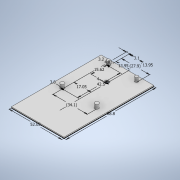
# Autodesk Inventor part: test fit for rfid reader
Saved by Autodesk Inventor 2020 (Build 240168000, 168)
## iProperties
Created: 2019-06-28
Part Number: test fit for rfid reader
Material: Generic
Document SubType Name: Modeling
Designer: jjsch
Density: 1 g/cm^3
Appearance: Default
Author: jjsch
Autodesk Inventor part; units mm, degrees
ref_plane "YZ Plane" through (0, 0, 0) normal (1, 0, 0) x (0, 1, 0)
ref_plane "XZ Plane" through (0, 0, 0) normal (0, 1, 0) x (-1, 0, 0)
ref_plane "XY Plane" through (0, 0, 0) normal (0, 0, 1) x (1, 0, 0)
sketch "Sketch1" plane through (0, 0, 0) normal (0, 1, 0) x (-1, 0, 0)
  point P0 (0, 0)
sketch "Sketch2" plane through (0, 0, 0) normal (0, 1, 0) x (-1, 0, 0)
  line L0 (0, 0) -> (-52.05, 0)
  line L1 (-52.05, 0) -> (-52.05, 88.8)
  line L2 (-52.05, 88.8) -> (0, 88.8)
  line L3 (0, 88.8) -> (0, 0)
  circle A0 centre (-8.975, 47.33) radius 1.9
  line L4 (-26.025, 67.1436) -> (-26.025, 88.8)
  circle A1 centre (-12.075, 4.83) radius 1.6
  circle A2 centre (-43.075, 47.33) radius 1.9
  circle A3 centre (-39.975, 4.83) radius 1.6
  circle A4 centre (-26.025, 20.45) radius 2
  dimension "d0" = 52.05
  dimension "d1" = 88.8
  dimension "d2" = 3.8
  dimension "d4" = 17.05
  dimension "d5" = 3.2
  dimension "d6" = 13.95
  dimension "d7" = 42.5
  dimension "d12" = 4.83
  dimension "d13" = 4
  dimension "d17" = 15.62
  dimension "d18" = 27.9
  dimension "d19" = 3.1
  dimension "d20" = 13.95
  constraints: 10 end point, 5 centre point, 2 parallel, 2 symmetric about line, 1 horizontal, 1 midpoint, 1 perpendicular, 2 other
  measures "d0" distance of L1.end L2.end
  measures "d1" distance of L0.end L1.end
  measures "d2" diameter of A0
  measures "d4" distance from line of L4 A0.centre
  measures "d5" diameter of A1
  measures "d6" distance from line of L4 A1.centre
  measures "d7" vertical distance of A1.centre A0.centre
  measures "d12" distance from line of L0 A1.centre
  measures "d13" diameter of A4
  measures "d17" vertical distance of A1.centre A4.centre
  measures "d18" distance of A3.centre A1.centre
  measures "d19" horizontal distance of A0.centre A1.centre
  measures "d20" horizontal distance of A4.centre A1.centre
extrude "Extrusion1" add sketch "Sketch2" along normal blind 5 contours A0 | A1 | A2 | A3
sketch "Sketch3" plane through (43.075, 0, 47.33) normal (0, -1, 0) x (1, 0, 0)
  circle A0 centre (0, 0) radius 1.9 projected
  circle A1 centre (-34.1, 0) radius 1.9 projected
  point P0 (-43.075, -47.33)
  dimension "d21" = 34.1
  measures "d21" distance of A0.centre A1.centre
extrude "Extrusion2" add sketch "Sketch2" along normal blind 1 contours L0 L1 L2 L3 | A4
extrude "Extrusion3" cut sketch "Sketch2" along normal mid plane 5 contours A4
body "Solid1"
